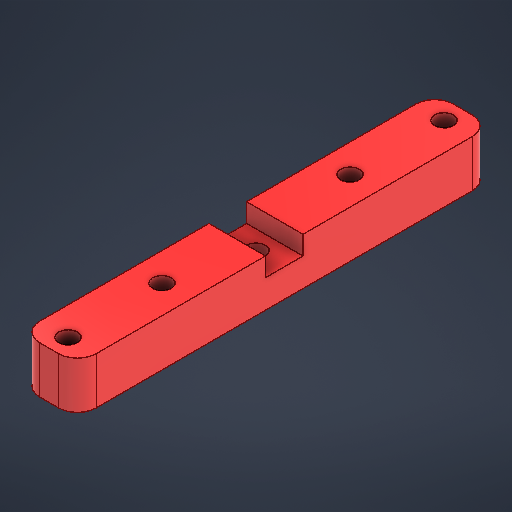
# Autodesk Inventor part: measuring_line
Saved by Autodesk Inventor 2026.1 (Build 301233000, 233)
## iProperties
Created: 2025-12-26
Part Number: measuring_line
Material: Generic
Document SubType Name: Modeling
Designer: emanuel
Density: 1 g/cm^3
Appearance: Light Red
Author: emanuel
Autodesk Inventor part; units mm, degrees
ref_plane "YZ Plane" through (0, 0, 0) normal (1, 0, 0) x (0, 1, 0)
ref_plane "XZ Plane" through (0, 0, 0) normal (0, 1, 0) x (-1, 0, 0)
ref_plane "XY Plane" through (0, 0, 0) normal (0, 0, 1) x (1, 0, 0)
sketch "Sketch1" plane through (0, 0, 0) normal (0, 1, 0) x (-1, 0, 0)
  circle A0 centre (0, 0) radius 1
  line L0 (0, 0) -> (3, 0)
  line L1 (3, 0) -> (3, 2)
  line L2 (3, 2) -> (0, 2)
  line L3 (0, 2) -> (0, 0)
  line L4 (3, 2) -> (-3, 2)
  line L5 (-3, 2) -> (-3, -2)
  line L6 (-3, -2) -> (3, -2)
  line L7 (3, -2) -> (3, 2)
  line L8 (3, -2) -> (-3, -2)
  line L9 (-3, -2) -> (-3, -22)
  line L10 (-3, -22) -> (3, -22)
  line L11 (3, -22) -> (3, -2)
  line L12 (3, 2) -> (-3, 2)
  line L13 (-3, 2) -> (-3, 22)
  line L14 (-3, 22) -> (3, 22)
  line L15 (3, 22) -> (3, 2)
  line L16 (0, 0) -> (0, 10)
  line L17 (0, 10) -> (0, 20)
  line L18 (0, 0) -> (0, -10)
  line L19 (0, -10) -> (0, -20)
  circle A1 centre (0, 20) radius 1
  circle A2 centre (0, 10) radius 1
  circle A3 centre (0, -10) radius 1
  circle A4 centre (0, -20) radius 1
  dimension "d0" = 2
  dimension "d1" = 3
  dimension "d2" = 2
  dimension "d3" = 6
  dimension "d4" = 4
  dimension "d5" = 20
  dimension "d6" = 6
  dimension "d7" = 20
  dimension "d8" = 10
  dimension "d9" = 10
  dimension "d10" = 10
  dimension "d11" = 10
  dimension "d12" = 2
  dimension "d13" = 2
  dimension "d14" = 2
  dimension "d15" = 2
  constraints: 40 end point, 8 parallel, 5 centre point, 5 coincident, 4 horizontal, 4 perpendicular, 3 point on line, 2 vertical
  measures "d0" diameter of A0
  measures "d1" distance of L2.end L1.end
  measures "d2" distance of L1.end L0.end
  measures "d3" distance of L6.end L5.end
  measures "d4" distance of L5.end L4.end
  measures "d5" distance of L9.end L8.end
  measures "d6" distance of L13.end L14.end
  measures "d7" distance of L12.end L13.end
  measures "d8" distance of L0.start L16.end
  measures "d9" distance of L16.end L17.end
  measures "d10" distance of L0.start L18.end
  measures "d11" distance of L18.end L19.end
  measures "d12" diameter of A1
  measures "d13" diameter of A2
  measures "d14" diameter of A3
  measures "d15" diameter of A4
extrude "Extrusion1" add sketch "Sketch1" along normal blind 2 contours L4 L13 L14 L15 L2 | L6 L11 L10 L9
extrude "Extrusion2" add sketch "Sketch1" against normal blind 3 contours L0 L7 L6 L18 A0 | A0 L3 L2 L1 L0 | A0 L18 L6 L5 L4 L3 | L4 L13 L14 L15 L2 | L6 L11 L10 L9
fillet "Fillet1" radius 2 4 edges at (3, -0.5, 22) (3, -0.5, -22) (-3, -0.5, -22) (-3, -0.5, 22)
body "Solid1"
